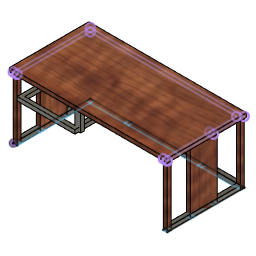
TABLE v2 (Autodesk Fusion 360 design; units mm, degrees)
Autodesk Fusion 360 part; units mm, degrees
sketch "Sketch1" plane through (0, 0, 0) normal (0, 0, 1) x (1, 0, 0)
  line L0 (0, 0) -> (0, 100)
  line L1 (0, 100) -> (200, 100)
  line L2 (200, 100) -> (200, 0)
  line L3 (200, 0) -> (195, 0)
  line L4 (195, 0) -> (195, 95)
  line L5 (195, 95) -> (5, 95)
  line L6 (5, 95) -> (5, 0)
  line L7 (5, 0) -> (0, 0)
  line L8 (0, 100) -> (5, 100)
  line L9 (5, 100) -> (5, 95)
  line L10 (5, 95) -> (0, 95)
  line L11 (0, 95) -> (0, 100)
  line L12 (200, 100) -> (195, 100)
  line L13 (195, 100) -> (195, 95)
  line L14 (195, 95) -> (200, 95)
  line L15 (200, 95) -> (200, 100)
  line L16 (195, 0) -> (200, 0)
  line L17 (200, 0) -> (200, 5)
  line L18 (200, 5) -> (195, 5)
  line L19 (195, 5) -> (195, 0)
  line L20 (0, 0) -> (5, 0)
  line L21 (5, 0) -> (5, 5)
  line L22 (5, 5) -> (0, 5)
  line L23 (0, 5) -> (0, 0)
  line L24 (50, 100) -> (55, 100)
  line L25 (55, 100) -> (55, 95)
  line L26 (55, 95) -> (50, 95)
  line L27 (50, 95) -> (50, 100)
  line L28 (150, 100) -> (145, 100)
  line L29 (145, 100) -> (145, 95)
  line L30 (145, 95) -> (150, 95)
  line L31 (150, 95) -> (150, 100)
  line L32 (195, 65) -> (200, 65)
  line L33 (200, 65) -> (200, 60)
  line L34 (200, 60) -> (195, 60)
  line L35 (195, 60) -> (195, 65)
  line L36 (195, 30) -> (200, 30)
  line L37 (200, 30) -> (200, 35)
  line L38 (200, 35) -> (195, 35)
  line L39 (195, 35) -> (195, 30)
  line L40 (0, 65) -> (5, 65)
  line L41 (5, 65) -> (5, 60)
  line L42 (5, 60) -> (0, 60)
  line L43 (0, 60) -> (0, 65)
  line L44 (0, 30) -> (5, 30)
  line L45 (5, 30) -> (5, 35)
  line L46 (5, 35) -> (0, 35)
  line L47 (0, 35) -> (0, 30)
  dimension "d1" = 100
  dimension "d2" = 200
  dimension "d3" = 5
  dimension "d4" = 95
  constraint coincident L0.start L7.end
  constraint vertical L0
  constraint perpendicular L0 L1
  constraint perpendicular L1 L2
  constraint perpendicular L2 L3
  constraint perpendicular L3 L4
  constraint perpendicular L4 L5
  constraint perpendicular L5 L6
  constraint perpendicular L6 L7
  constraint horizontal L8
  constraint vertical L9
  constraint horizontal L10
  constraint vertical L11
  constraint horizontal L12
  constraint vertical L13
  constraint horizontal L14
  constraint vertical L15
  constraint horizontal L16
  constraint vertical L17
  constraint horizontal L18
  constraint vertical L19
  constraint coincident L2 L17.end
  constraint horizontal L20
  constraint vertical L21
  constraint horizontal L22
  constraint vertical L23
  constraint horizontal L24
  constraint vertical L25
  constraint horizontal L26
  constraint vertical L27
  constraint coincident L5 L25.end
  constraint coincident L1 L24.start
  constraint horizontal L28
  constraint vertical L29
  constraint horizontal L30
  constraint vertical L31
  constraint coincident L1 L28.start
  constraint horizontal L32
  constraint vertical L33
  constraint horizontal L34
  constraint vertical L35
  constraint coincident L4 L32.start
  constraint horizontal L36
  constraint vertical L37
  constraint horizontal L38
  constraint vertical L39
  constraint coincident L4 L36.start
  constraint horizontal L40
  constraint vertical L41
  constraint horizontal L42
  constraint vertical L43
  constraint coincident L6 L41.end
  constraint coincident L0 L40.start
  constraint horizontal L44
  constraint vertical L45
  constraint horizontal L46
  constraint vertical L47
  constraint coincident L0 L44.start
  measures "d1" distance of L0.start L0.end
  measures "d2" distance of L0.end L1.end
  measures "d3" distance of L2.end L3.end
  measures "d4" distance of L3.end L4.end
extrude "Extrude1" add sketch "Sketch1" along normal blind 80 contours L0 L1 L8 L9 L10 L11 makes body 1
extrude "Extrude2" add sketch "Sketch1" along normal blind 80 separate body contours L1 L2 L12 L13 L14 L15 makes body 2
extrude "Extrude3" add sketch "Sketch1" along normal blind 80 separate body contours L0 L6 L7 L20 L21 L22 L23 makes body 3
extrude "Extrude4" add sketch "Sketch1" along normal blind 80 separate body contours L2 L3 L4 L16 L17 L18 L19 makes body 4
extrude "Extrude5" add sketch "Sketch1" along normal blind 5 separate body contours L0 L6 L22 L44 | L0 L6 L44 L45 L46 L47 | L0 L6 L42 L46 | L0 L6 L40 L41 L42 L43 | L0 L6 L10 L40 | L1 L5 L9 L27 | L1 L5 L24 L25 L26 L27 | L1 L5 L25 L29 | L1 L5 L28 L29 L30 L31 | L1 L5 L13 L31 | L2 L4 L14 L32 | L2 L4 L32 L33 L34 L35 | L2 L4 L34 L38 | L2 L4 L36 L37 L38 L39 | L2 L4 L18 L36 makes body 5
extrude "Extrude6" add sketch "Sketch1" along normal blind 80 separate body contours L1 L5 L24 L25 L26 L27 makes body 6
extrude "Extrude7" add sketch "Sketch1" along normal blind 80 separate body contours L1 L5 L28 L29 L30 L31 makes body 7
extrude "Extrude8" add sketch "Sketch1" along normal blind 80 separate body contours L1 L5 L25 L29 makes body 8
extrude "Extrude9" add sketch "Sketch1" along normal blind 80 separate body contours L0 L6 L40 L41 L42 L43 makes body 9
extrude "Extrude10" add sketch "Sketch1" along normal blind 80 separate body contours L0 L6 L44 L45 L46 L47 makes body 10
extrude "Extrude11" add sketch "Sketch1" along normal blind 80 separate body contours L2 L4 L32 L33 L34 L35 makes body 11
extrude "Extrude12" add sketch "Sketch1" along normal blind 80 separate body contours L2 L4 L36 L37 L38 L39 makes body 12
extrude "Extrude13" add sketch "Sketch1" along normal blind 80 separate body contours L0 L6 L42 L46 makes body 13
extrude "Extrude14" add sketch "Sketch1" along normal blind 80 separate body contours L2 L4 L34 L38 makes body 14
ref_plane "WorkPlane2" through (2.5, 97.5, 80) normal (0, 0, 1) x (1, 0, 0)
sketch "Sketch2" plane through (0, 0, 0) normal (0, 0, 1) x (1, 0, 0)
  line L0 (0, 100) -> (200, 100)
  line L1 (195, 95) -> (5, 95)
  line L2 (5, 95) -> (5, 0)
  line L3 (0, 0) -> (0, 100)
  line L4 (195, 0) -> (195, 95)
  line L5 (200, 100) -> (200, 0)
  line L6 (200, 0) -> (195, 0)
  line L7 (0, 0) -> (5, 0)
sketch "Sketch3" plane through (2.5, 97.5, 80) normal (0, 0, 1) x (1, 0, 0)
  line L0 (192.5, -2.5) -> (2.5, -2.5)
  line L1 (2.5, -2.5) -> (2.5, -97.5)
  line L2 (197.5, 2.5) -> (197.5, -97.5)
  line L3 (197.5, -37.5) -> (192.5, -37.5)
  line L4 (192.5, -97.5) -> (192.5, -2.5)
  line L5 (-2.5, 2.5) -> (197.5, 2.5)
  line L6 (-2.5, -97.5) -> (-2.5, 2.5)
  line L7 (2.5, -97.5) -> (-2.5, -97.5)
  line L8 (197.5, -97.5) -> (192.5, -97.5)
box "BoxPrimitive1" add length 103.072 width 205 height 5 placed x (0, -1, 0) y (1, 0, 0) z (0, 0, 1) at (-2.5, 100.572, 80) bodies 1 5 2 3 4 6 7 8 9 10 11 12 13 14
ref_plane "WorkPlane4" through (100, 50, 50) normal (0, 0, 1) x (1, 0, 0)
sketch "Sketch5" plane through (100, 50, 50) normal (0, 0, 1) x (1, 0, 0)
  line L0 (20, -110) -> (0, -70)
  line L1 (-95, -50) -> (-20, -50)
  line L2 (-20, -50) -> (-20, 45)
  line L3 (-20, 45) -> (-25, 45)
  line L4 (-25, 45) -> (-25, -45)
  line L5 (-25, -45) -> (-90, -45)
  line L6 (-90, -45) -> (-90, 45)
  line L7 (-90, 45) -> (-20, 45)
  line L8 (-95, -50) -> (-95, 45)
  line L9 (-95, 45) -> (-90, 45)
  dimension "d42" = 75
  constraint horizontal L1
  constraint perpendicular L1 L2
  constraint perpendicular L2 L3
  constraint perpendicular L3 L4
  constraint perpendicular L2 L5
  constraint perpendicular L3 L6
  constraint perpendicular L2 L7
  constraint perpendicular L1 L8
  constraint perpendicular L6 L9
  measures "d42" distance of L1.start L1.end
extrude "Extrude15" add sketch "Sketch5" along normal blind 5 separate body contours L1 L2 L3 L4 L5 L6 L7 L8 L9 makes body 15
ref_plane "WorkPlane6" through (42.5, 0, 52.5) normal (0, -1, 0) x (1, 0, 0)
sketch "Sketch6" plane through (42.5, 0, 52.5) normal (0, -1, 0) x (1, 0, 0)
  line L0 (30, 0) -> (30, 40)
  line L1 (30, 40) -> (35, 40)
  line L2 (35, 40) -> (35, 0)
  line L3 (35, 0) -> (30, 0)
  constraint vertical L0
  constraint perpendicular L0 L1
  constraint perpendicular L1 L2
  constraint perpendicular L0 L3
extrude "Extrude16" add sketch "Sketch6" against normal blind 5 separate body makes body 16
move_face "MoveFace1" by (1.7004, 0.0606, 0.2791) 1 faces at (74.1667, 0, 65.8333) on bodies 16
move_body "Move1" bodies 16 to x (1, 0, 0) y (0, 1, 0) z (0, 0, 1) at (2.2702, -0.3816, -2.2327)
move_face "MoveFace2" by (1.9842, 0, -29.8187) 1 faces at (76.4368, -0.321, 63.6006) on bodies 16
delete_body "RemoveBody1" bodies 16
ref_plane "WorkPlane7" through (42.5, 0, 52.5) normal (0, -1, 0) x (1, 0, 0)
sketch "Sketch7" plane through (0, 0, 0) normal (0, -1, 0) x (1, 0, 0)
  line L0 (5, 50) -> (80, 50)
  line L1 (80, 50) -> (80, 55)
  line L2 (80, 55) -> (5, 55)
  line L3 (5, 55) -> (5, 50)
  line L4 (75, 50, -5) -> (80, 50, -5)
  line L5 (80, 50, -5) -> (80, 80, -5)
  line L6 (80, 80, -5) -> (75, 80, -5)
  line L7 (75, 80, -5) -> (75, 50, -5)
  point P0 (75, 50)
extrude "Extrude17" add sketch "Sketch7" against normal blind 5 separate body contours L4 L5 L6 L7 in plane through (0, 5, 0) normal (0, -1, 0) makes body 17
move_face "MoveFace3" by (2.43, -11.9116, 8.3999) 1 faces at (80, 6.6667, 60) on bodies 17
move_face "MoveFace4" by (0, -5, 0) 1 faces at (82.43, 6.6667, 60) on bodies 17
